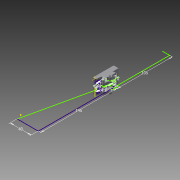
# Autodesk Inventor part: clip_hinge(2)
Saved by Autodesk Inventor 2015 (Build 190159000, 159)
## iProperties
Created: 2017-10-02
Part Number: clip_hinge(2)
Material: Generic
Document SubType Name: Modeling
Designer: Anshul
Density: 1 g/cm^3
Appearance: Default
Author: Anshul
Autodesk Inventor part; units mm, degrees
note: some values were not read from the file. Chosen so that the rebuilt part matches the saved one: arc direction of "Extrusion4".
ref_plane "YZ Plane" through (0, 0, 0) normal (1, 0, 0) x (0, 1, 0)
ref_plane "XZ Plane" through (0, 0, 0) normal (0, 1, 0) x (-1, 0, 0)
ref_plane "XY Plane" through (0, 0, 0) normal (0, 0, 1) x (1, 0, 0)
sketch "Sketch1" plane through (0, 0, 0) normal (0, 1, 0) x (-1, 0, 0)
  line L0 (0, 0) -> (0, -145)
  line L1 (0, -145) -> (3, -145)
  line L2 (3, -145) -> (8, -145)
  circle A0 centre (8, -145) radius 1.5
  line L3 (0, 0) -> (40, 0)
  line L4 (0, -145) -> (0, -250)
  line L5 (0, -250) -> (8, -250)
  line L6 (8, -156) -> (8, -148)
  circle A1 centre (8, -145) radius 3
  line L7 (13, -250) -> (8, -250)
  line L8 (8, -156) -> (13, -156)
  line L9 (13, -156) -> (13, -166)
  line L10 (10.3705, -134.2585) -> (15.1383, -135.3107)
  line L11 (15.1383, -135.3107) -> (14.892, -136.4268)
  line L12 (15.1383, -135.3107) -> (17.2934, -125.5456)
  line L13 (17.2934, -125.5456) -> (12.5256, -124.4934)
  line L14 (17.2934, -125.5456) -> (22.1759, -126.6232)
  line L15 (13, -166) -> (18, -166)
  line L16 (22.1759, -126.6232) -> (22.1759, -166)
  line L17 (22.1759, -166) -> (18, -166)
  arc A2 (0, -137.4502) -> (0, -152.5498) centre (8, -145) ccw
  arc A3 (8, -156) -> (10.3705, -134.2585) centre (8, -145) ccw
  line L18 (40, 0) -> (12.5256, -124.4934)
  line L19 (10.3705, -134.2585) -> (8.6465, -142.0705)
  line L20 (8, -148) -> (8, -153)
  arc A4 (0, -142.1277) -> (0, -147.8723) centre (8, -145) ccw
  arc A5 (8, -153.5) -> (9.8318, -136.6997) centre (8, -145) ccw
  line L21 (8, -153.5) -> (8, -156)
  line L22 (9.8318, -136.6997) -> (10.3705, -134.2585)
  line L23 (9.5, -145) -> (11.2347, -137.1396)
  line L24 (9.5, -145) -> (16.5, -145)
  line L25 (13, -156) -> (13, -154.798)
  line L26 (16.5, -145) -> (19, -145)
  line L27 (11.2347, -137.1396) -> (11.7798, -134.6698)
  dimension "d4" = 3
  dimension "d0" = 145
  dimension "d1" = 3
  dimension "d2" = 5
  dimension "d5" = 40
  dimension "d6" = 105
  dimension "d8" = 6
  dimension "d10" = 10
  dimension "d11" = 10
  dimension "d12" = 5
  dimension "d13" = 5
  constraints: 56 end point, 16 point on circle, 12 perpendicular, 10 point on line, 5 centre point, 3 collinear, 2 coincident, 2 horizontal, 2 parallel, 2 tangent, 1 horizontal alignment, 1 vertical, 2 other
  measures "d0" distance of L0.start L0.end
  measures "d1" distance of L0.end L1.end
  measures "d2" distance of L1.end L2.end
  measures "d5" distance of L0.start L3.end
  measures "d6" distance of L0.end L4.end
  measures "d8" diameter of A1
  measures "d10" distance of L8.end L9.end
  measures "d11" distance of L10.end L12.end
  measures "d12" distance of L12.end L14.end
  measures "d13" distance of L9.end L15.end
extrude "Extrusion4" add sketch "Sketch1" along normal mid plane 28 contours L14 L16 L17 L15 L9 L25 A3 L11 L12 | A1 L23 A0 L2 | L2 A0 L24 A1 | A3 L27 A5 L19 | A3 L26 A5 L27 | L19 A5 L23 A1 | A1 L24 A5 L6 | A3 L6 A5 L26 | L23 A1 L24 | L23 A5 L24 A1
extrude "Extrusion5" cut sketch "Sketch1" along normal mid plane 18.5 contours A1 L23 A0 L2 | L2 A0 L24 A1 | L19 A5 L23 A1 | A1 L24 A5 L6 | L23 A1 L24 | L23 A5 L24 A1
extrude "Extrusion6" cut sketch "Sketch1" along normal mid plane 10.5 contours A3 L27 A5 L19 | A3 L26 A5 L27 | A3 L6 A5 L26
extrude "Extrusion7" add sketch "Sketch1" along normal mid plane 9.5 contours A3 L26 A5 L27 | L23 A1 L24 | L23 A5 L24 A1
sketch "Sketch2" plane through (-17.2934, -14, -125.5456) normal (0.9765029, 0, 0.2155041) x (0.2155041, 0, -0.9765029)
  line L0 (0, 28) -> (0, 14)
  line L1 (0, 0) -> (0, 28) projected
  line L2 (0, 14) -> (5, 14)
  line L3 (5, 14) -> (5, 21)
  line L4 (5, 14) -> (5, 7)
  circle A0 centre (5, 21) radius 2.4
  circle A1 centre (5, 7) radius 2.4
  circle A2 centre (5, 21) radius 4
  circle A3 centre (5, 7) radius 4
  point P0 (-118.8689, 14)
  dimension "d29" = 5
  dimension "d30" = 7
  dimension "d31" = 7
  dimension "d32" = 4.8
  dimension "d33" = 4.8
  dimension "d34" = 8
  dimension "d35" = 8
  constraints: 8 end point, 4 centre point, 4 coincident, 1 horizontal, 1 midpoint, 1 perpendicular, 1 point on line
  measures "d29" distance of L0.end L2.end
  measures "d30" distance of L2.end L3.end
  measures "d31" distance of L2.end L4.end
  measures "d32" diameter of A0
  measures "d33" diameter of A1
  measures "d34" diameter of A2
  measures "d35" diameter of A3
extrude "Extrusion8" cut sketch "Sketch2" against normal blind 10.5 contours A0 | A1 | A2 | A3
extrude "Extrusion9" add sketch "Sketch2" against normal blind 5
sketch "Sketch3" plane through (-13, -14, -166) normal (1, 0, 0) x (0, 0, -1)
  line L0 (0, 28) -> (0, 14)
  line L1 (0, 0) -> (0, 28) projected
  line L2 (0, 14) -> (-5, 14)
  line L3 (-5, 14) -> (-5, 21)
  line L4 (-5, 14) -> (-5, 7)
  circle A0 centre (-5, 21) radius 2.4
  circle A1 centre (-5, 7) radius 2.4
  point P0 (-166, 14)
  dimension "d40" = 5
  dimension "d41" = 7
  dimension "d42" = 7
  dimension "d43" = 4.8
  dimension "d44" = 4.8
  constraints: 8 end point, 2 centre point, 2 coincident, 2 perpendicular, 1 midpoint, 1 point on line
  measures "d40" distance of L0.end L2.end
  measures "d41" distance of L2.end L3.end
  measures "d42" distance of L2.end L4.end
  measures "d43" diameter of A0
  measures "d44" diameter of A1
extrude "Extrusion10" cut sketch "Sketch3" against normal blind 10
body "Solid2"
